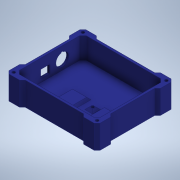
# Autodesk Inventor part: Case
Saved by Autodesk Inventor 2020 (Build 240168000, 168)
## iProperties
Created: 2020-02-03
Part Number: Case
Material: Generic
Document SubType Name: Modeling
Designer: Alex
Density: 1 g/cm^3
Appearance: Default
Author: Alex
Autodesk Inventor part; units mm, degrees
ref_plane "YZ Plane" through (0, 0, 0) normal (1, 0, 0) x (0, 1, 0)
ref_plane "XZ Plane" through (0, 0, 0) normal (0, 1, 0) x (-1, 0, 0)
ref_plane "XY Plane" through (0, 0, 0) normal (0, 0, 1) x (1, 0, 0)
sketch "Sketch1" plane through (0, 0, 0) normal (0, 1, 0) x (-1, 0, 0)
  line L0 (-60, 50) -> (-41, 50) construction
  line L1 (60, 50) -> (60, 31) construction
  line L2 (60, -50) -> (41, -50) construction
  line L3 (-60, -50) -> (-60, -31) construction
  line L4 (-60, 50) -> (60, -50) construction
  line L5 (60, 50) -> (-60, -50) construction
  line L6 (41, -50) -> (45, -54)
  line L7 (45, -54) -> (60, -54)
  line L8 (60, -54) -> (64, -50)
  line L9 (64, -50) -> (64, -35)
  line L10 (64, -35) -> (60, -31)
  line L11 (-41, -50) -> (-45, -54)
  line L12 (-45, -54) -> (-60, -54)
  line L13 (-60, -54) -> (-64, -50)
  line L14 (-64, -50) -> (-64, -35)
  line L15 (-64, -35) -> (-60, -31)
  line L16 (-60, 31) -> (-64, 35)
  line L17 (-64, 35) -> (-64, 50)
  line L18 (-64, 50) -> (-60, 54)
  line L19 (-60, 54) -> (-45, 54)
  line L20 (-45, 54) -> (-41, 50)
  line L21 (41, 50) -> (45, 54)
  line L22 (45, 54) -> (60, 54)
  line L23 (60, 54) -> (64, 50)
  line L24 (64, 50) -> (64, 35)
  line L25 (64, 35) -> (60, 31)
  line L26 (41, -50) -> (-41, -50)
  line L27 (60, -31) -> (60, -50) construction
  line L28 (60, 31) -> (60, -31)
  line L29 (41, 50) -> (60, 50) construction
  line L30 (-41, 50) -> (41, 50)
  line L31 (-60, 31) -> (-60, 50) construction
  line L32 (-41, -50) -> (-60, -50) construction
  line L33 (-60, -31) -> (-60, 31)
  point P0 (0, 0)
  point P1 (0, 0)
  point P2 (0, 0)
  dimension "d4" = 120
  dimension "d5" = 100
  dimension "d6" = 45
  dimension "d7" = 15
  dimension "d8" = 4
  dimension "d9" = 4
  dimension "d12" = 45
  dimension "d13" = 4
  constraints: 68 end point, 21 parallel, 16 perpendicular, 7 equal length, 6 collinear, 6 vertical alignment, 5 horizontal, 3 horizontal alignment, 3 midpoint, 1 coincident, 1 point on line
  measures "d4" distance of L2.start L3.start
  measures "d5" distance of L1.start L2.start
  measures "d6" angle of L6 L2
  measures "d7" distance of L6.end L7.end
  measures "d8" distance between parallel lines of L7 L2
  measures "d9" horizontal distance of L7.end L8.end
  measures "d12" angle of L2 L11
  measures "d13" distance between parallel lines of L14 L3
extrude "Extrusion2" add sketch "Sketch1" along normal blind 3
sketch "Sketch2" plane through (0, 3, 0) normal (0, 1, 0) x (1, 0, 0)
  line L0 (-64, 50) -> (-64, 35) projected
  line L1 (-64, 35) -> (-60, 31) projected
  line L2 (-60, 31) -> (-60, -31) projected
  line L3 (-60, -31) -> (-64, -35) projected
  line L4 (-64, -35) -> (-64, -50) projected
  line L5 (-64, -50) -> (-60, -54) projected
  line L6 (-60, -54) -> (-45, -54) projected
  line L7 (-45, -54) -> (-41, -50) projected
  line L8 (-41, -50) -> (41, -50) projected
  line L9 (41, -50) -> (45, -54) projected
  line L10 (45, -54) -> (60, -54) projected
  line L11 (60, -54) -> (64, -50) projected
  line L12 (64, -50) -> (64, -35) projected
  line L13 (64, -35) -> (60, -31) projected
  line L14 (60, -31) -> (60, 31) projected
  line L15 (60, 31) -> (64, 35) projected
  line L16 (64, 35) -> (64, 50) projected
  line L17 (64, 50) -> (60, 54) projected
  line L18 (60, 54) -> (45, 54) projected
  line L19 (45, 54) -> (41, 50) projected
  line L20 (41, 50) -> (-41, 50) projected
  line L21 (-41, 50) -> (-45, 54) projected
  line L22 (-45, 54) -> (-60, 54) projected
  line L23 (-60, 54) -> (-64, 50) projected
  line L24 (-42.2426, 47) -> (42.2426, 47)
  line L25 (42.2426, 47) -> (46.2426, 51) construction
  line L26 (46.2426, 51) -> (58.7574, 51) construction
  line L27 (58.7574, 51) -> (61, 48.7574) construction
  line L28 (61, 48.7574) -> (61, 36.2426) construction
  line L29 (61, 36.2426) -> (57, 32.2426) construction
  line L30 (57, 32.2426) -> (57, -32.2426)
  line L31 (57, -32.2426) -> (61, -36.2426) construction
  line L32 (61, -36.2426) -> (61, -48.7574) construction
  line L33 (61, -48.7574) -> (58.7574, -51) construction
  line L34 (58.7574, -51) -> (46.2426, -51) construction
  line L35 (46.2426, -51) -> (42.2426, -47) construction
  line L36 (42.2426, -47) -> (-42.2426, -47)
  line L37 (-42.2426, -47) -> (-46.2426, -51) construction
  line L38 (-46.2426, -51) -> (-58.7574, -51) construction
  line L39 (-58.7574, -51) -> (-61, -48.7574) construction
  line L40 (-61, -48.7574) -> (-61, -36.2426) construction
  line L41 (-61, -36.2426) -> (-57, -32.2426) construction
  line L42 (-57, -32.2426) -> (-57, 32.2426)
  line L43 (-57, 32.2426) -> (-61, 36.2426) construction
  line L44 (-61, 36.2426) -> (-61, 48.7574) construction
  line L45 (-61, 48.7574) -> (-58.7574, 51) construction
  line L46 (-58.7574, 51) -> (-46.2426, 51) construction
  line L47 (-46.2426, 51) -> (-42.2426, 47) construction
  line L48 (-42.2426, 47) -> (-52.2426, 47)
  line L49 (-52.2426, 47) -> (-57, 42.2426)
  line L50 (-57, 42.2426) -> (-57, 32.2426)
  line L51 (-57, -32.2426) -> (-57, -42.2426)
  line L52 (-57, -42.2426) -> (-52.2426, -47)
  line L53 (-52.2426, -47) -> (-42.2426, -47)
  line L54 (42.2426, -47) -> (52.2426, -47)
  line L55 (52.2426, -47) -> (57, -42.2426)
  line L56 (57, -42.2426) -> (57, -32.2426)
  line L57 (57, 32.2426) -> (57, 42.2426)
  line L58 (57, 42.2426) -> (52.2426, 47)
  line L59 (52.2426, 47) -> (42.2426, 47)
  point P0 (0, 0)
  dimension "d16" = 3
  dimension "d17" = 10
  constraints: 72 end point, 7 equal length, 4 perpendicular, 2 point on line, 1 horizontal, 1 vertical, 23 other
  measures "d16" distance between parallel lines of L20 L24
  measures "d17" distance of L24.start L48.end
extrude "Extrusion3" add sketch "Sketch2" along normal blind 30
sketch "Sketch4" plane through (0, 3, 0) normal (0, 1, 0) x (1, 0, 0)
  line L0 (45, 54) -> (41, 50) construction
  line L1 (41, 50) -> (-41, 50) construction
  line L2 (-41, 50) -> (-45, 54) construction
  line L3 (-45, 54) -> (-60, 54) construction
  line L4 (-60, 54) -> (-64, 50) construction
  line L5 (-64, 50) -> (-64, 35) construction
  line L6 (-64, 35) -> (-60, 31) construction
  line L7 (-60, 31) -> (-60, -31) construction
  line L8 (-60, -31) -> (-64, -35) construction
  line L9 (-64, -35) -> (-64, -50) construction
  line L10 (-64, -50) -> (-60, -54) construction
  line L11 (-60, -54) -> (-45, -54) construction
  line L12 (-45, -54) -> (-41, -50) construction
  line L13 (-41, -50) -> (41, -50) construction
  line L14 (41, -50) -> (45, -54) construction
  line L15 (45, -54) -> (60, -54) construction
  line L16 (60, -54) -> (64, -50) construction
  line L17 (64, -50) -> (64, -35) construction
  line L18 (64, -35) -> (60, -31) construction
  line L19 (60, -31) -> (60, 31) construction
  line L20 (60, 31) -> (64, 35) construction
  line L21 (64, 35) -> (64, 50) construction
  line L22 (64, 50) -> (60, 54) construction
  line L23 (60, 54) -> (45, 54) construction
  line L24 (-52.2426, 47) -> (52.2426, 47) construction
  line L25 (52.2426, 47) -> (57, 42.2426) construction
  line L26 (57, 42.2426) -> (57, -42.2426) construction
  line L27 (57, -42.2426) -> (52.2426, -47) construction
  line L28 (52.2426, -47) -> (-52.2426, -47) construction
  line L29 (-52.2426, -47) -> (-57, -42.2426) construction
  line L30 (-57, -42.2426) -> (-57, 42.2426) construction
  line L31 (-57, 42.2426) -> (-52.2426, 47) construction
  line L32 (-52.2426, 47) -> (-57, 42.2426) construction
  line L33 (-57, 42.2426) -> (-57, -42.2426) construction
  line L34 (-57, -42.2426) -> (-52.2426, -47) construction
  line L35 (-52.2426, -47) -> (52.2426, -47) construction
  line L36 (52.2426, -47) -> (57, -42.2426) construction
  line L37 (57, -42.2426) -> (57, 42.2426) construction
  line L38 (57, 42.2426) -> (52.2426, 47) construction
  line L39 (52.2426, 47) -> (-52.2426, 47) construction
  line L40 (-54, 9.34) -> (47.6, 9.34) construction
  line L41 (47.6, 9.34) -> (47.6, -44) construction
  line L42 (47.6, -44) -> (-54, -44) construction
  line L43 (-54, -44) -> (-54, 9.34) construction
  line L44 (9.6, -6) -> (14.6, -6)
  line L45 (14.6, -6) -> (14.6, -11)
  line L46 (14.6, -11) -> (9.6, -11)
  line L47 (9.6, -11) -> (9.6, -6)
  line L48 (9.6, -6) -> (14.6, -11) construction
  line L49 (14.6, -6) -> (9.6, -11) construction
  line L50 (45.02, -44) -> (40.02, -44)
  line L51 (40.02, -44) -> (40.02, -39)
  line L52 (40.02, -39) -> (45.02, -39)
  line L53 (45.02, -39) -> (45.02, -44)
  line L54 (45.02, -44) -> (40.02, -39) construction
  line L55 (40.02, -44) -> (45.02, -39) construction
  line L56 (-24, -0.66) -> (-4, -0.66)
  line L57 (-4, -0.66) -> (-4, -34)
  line L58 (-4, -34) -> (-24, -34)
  line L59 (-24, -34) -> (-24, -0.66)
  line L60 (21, -0.66) -> (31, -0.66)
  line L61 (31, -0.66) -> (31, -34)
  line L62 (31, -34) -> (21, -34)
  line L63 (21, -34) -> (21, -0.66)
  point P0 (-40, -41.5)
  point P1 (-38.7, 6.7)
  point P2 (12.1, -36.4)
  point P3 (12.1, -8.5)
  point P4 (36.2, 6.7)
  point P5 (42.52, -41.5)
  dimension "d20" = 53.34
  dimension "d21" = 101.6
  dimension "d23" = 3
  dimension "d24" = 3
  dimension "d25" = 14
  dimension "d26" = 1.3
  dimension "d27" = 50.8
  dimension "d29" = 2.5
  dimension "d30" = 5.1
  dimension "d31" = 27.9
  dimension "d32" = 15.2
  dimension "d33" = 24.1
  dimension "d34" = 96.52
  dimension "d35" = 30
  dimension "d36" = 50
  dimension "d37" = 10
  dimension "d38" = 10
  dimension "d39" = 75
  dimension "d40" = 85
  dimension "d41" = 5
  constraints: 48 end point, 10 parallel, 5 horizontal, 5 perpendicular, 4 midpoint, 3 equal length, 2 collinear, 2 horizontal alignment, 1 vertical alignment
  measures "d20" distance of L40.end L41.end
  measures "d21" distance of L40.start L40.end
  measures "d23" distance between parallel lines of L42 L28
  measures "d24" distance between parallel lines of L30 L43
  measures "d25" distance from line of point (-40, -41.5) L43
  measures "d26" horizontal distance of point (-38.7, 6.7) point (-40, -41.5)
  measures "d27" horizontal distance of point (12.1, -8.5) point (-38.7, 6.7)
  measures "d29" distance from line of point (42.52, -41.5) L42
  measures "d30" vertical distance of point (12.1, -36.4) point (-40, -41.5)
  measures "d31" distance of point (12.1, -8.5) point (12.1, -36.4)
  measures "d32" vertical distance of point (36.2, 6.7) point (12.1, -8.5)
  measures "d33" horizontal distance of point (36.2, 6.7) point (12.1, -8.5)
  measures "d34" distance from line of point (42.52, -41.5) L43
  measures "d35" distance between parallel lines of L59 L43
  measures "d36" distance between parallel lines of L57 L43
  measures "d37" distance between parallel lines of L56 L40
  measures "d38" distance between parallel lines of L58 L42
  measures "d39" distance between parallel lines of L63 L43
  measures "d40" distance between parallel lines of L61 L43
  measures "d41" distance of L45.end L46.end
extrude "Extrusion4" add sketch "Sketch4" along normal blind 3
chamfer "Chamfer1" distance 3 angle 45 16 edges at (-14, 3, 34) (-4, 3, 17.33) (21, 3, 17.33) (-24, 3, 17.33) (26, 3, 34) (40.02, 3, 41.5) (42.52, 3, 39) (45.02, 3, 41.5) (42.52, 3, 44) (9.6, 3, 8.5) (12.1, 3, 11) (14.6, 3, 8.5) (12.1, 3, 6) (26, 3, 0.66) (-14, 3, 0.66) (31, 3, 17.33)
sketch "Sketch5" plane through (0, 6, 0) normal (0, 1, 0) x (1, 0, 0)
  line L0 (14.6, -11) -> (14.6, -6) construction
  line L1 (14.6, -6) -> (9.6, -6) construction
  line L2 (9.6, -6) -> (9.6, -11) construction
  line L3 (9.6, -11) -> (14.6, -11) construction
  line L4 (40.02, -44) -> (45.02, -44) construction
  line L5 (45.02, -44) -> (45.02, -39) construction
  line L6 (45.02, -39) -> (40.02, -39) construction
  line L7 (40.02, -39) -> (40.02, -44) construction
  point P0 (0, 0)
  point P1 (12.1, -8.5)
  point P2 (42.52, -41.5)
  point P3 (14.6, -8.5)
  point P4 (45.02, -41.5)
  point P5 (12.1, -6)
  point P6 (42.52, -39)
  constraints: 4 midpoint, 2 horizontal alignment, 2 vertical alignment
hole "Hole1" at (12.1, 6, 8.5) at (42.52, 6, 41.5) direction (0, -1, 0) diameter 4 depth 5
sketch "Sketch6" plane through (-57, 3, 42.2426) normal (1, 0, 0) x (0, 0, -1)
  line L0 (44.5826, 0) -> (5.2426, 0) construction
  line L1 (5.2426, 0) -> (44.5826, 0) construction
  line L2 (5.2426, 0) -> (44.5826, 0) construction
  line L3 (44.5826, 0) -> (5.2426, 0) construction
  line L4 (-4.7574, 0) -> (6.2426, 0) construction
  line L5 (-4.7574, 0) -> (0, 0) construction
  line L6 (0, 0) -> (84.4853, 0) construction
  line L7 (84.4853, 0) -> (89.2426, 0) construction
  line L8 (89.2426, 0) -> (84.4853, 0) construction
  line L9 (84.4853, 0) -> (0, 0) construction
  line L10 (0, 0) -> (-4.7574, 0) construction
  line L11 (6.2426, 0) -> (-4.7574, 0) construction
  line L12 (39.2426, 0) -> (28.2426, 0) construction
  line L13 (28.2426, 0) -> (39.2426, 0) construction
  line L14 (-1.7574, 0) -> (51.5826, 0) construction
  line L15 (41.5826, 3) -> (8.2426, 3) construction
  line L16 (8.2426, 3) -> (41.5826, 3) construction
  line L17 (41.5826, 3) -> (44.5826, 0) construction
  line L18 (44.5826, 0) -> (41.5826, 3) construction
  line L19 (8.2426, 3) -> (5.2426, 0) construction
  line L20 (8.2426, 3) -> (5.2426, 0) construction
  line L21 (84.4853, 0) -> (0, 0) construction
  line L22 (84.4853, 0) -> (84.4853, 30) construction
  line L23 (0, 30) -> (84.4853, 30) construction
  line L24 (0, 0) -> (0, 30) construction
  line L25 (29.8326, 16.2) -> (42.3326, 16.2)
  line L26 (42.3326, 16.2) -> (42.3326, 4.7)
  line L27 (42.3326, 4.7) -> (29.8326, 4.7)
  line L28 (29.8326, 4.7) -> (29.8326, 16.2)
  point P0 (42.2426, -3)
  dimension "d55" = 11.5
  dimension "d56" = 12.5
  dimension "d57" = 1.7
  dimension "d58" = 9.25
  constraints: 8 end point, 2 parallel, 1 horizontal, 1 perpendicular, 1 other
  measures "d55" distance between parallel lines of L25 L27
  measures "d56" distance between parallel lines of L26 L28
  measures "d57" distance between parallel lines of L27 L15
  measures "d58" distance from line of point (51.583, 0) L26
extrude "Extrusion5" cut sketch "Sketch6" against normal blind 10
sketch "Sketch7" plane through (0, 33, 0) normal (0, 1, 0) x (1, 0, 0)
  line L0 (41, -50) -> (45, -54) construction
  line L1 (45, -54) -> (60, -54) construction
  line L2 (60, -54) -> (64, -50) construction
  line L3 (64, -50) -> (64, -35) construction
  line L4 (64, -35) -> (60, -31) construction
  line L5 (60, -31) -> (60, 31) construction
  line L6 (60, 31) -> (64, 35) construction
  line L7 (64, 35) -> (64, 50) construction
  line L8 (64, 50) -> (60, 54) construction
  line L9 (60, 54) -> (45, 54) construction
  line L10 (45, 54) -> (41, 50) construction
  line L11 (41, 50) -> (-41, 50) construction
  line L12 (-41, 50) -> (-45, 54) construction
  line L13 (-45, 54) -> (-60, 54) construction
  line L14 (-60, 54) -> (-64, 50) construction
  line L15 (-64, 50) -> (-64, 35) construction
  line L16 (-64, 35) -> (-60, 31) construction
  line L17 (-60, 31) -> (-60, -31) construction
  line L18 (-60, -31) -> (-64, -35) construction
  line L19 (-64, -35) -> (-64, -50) construction
  line L20 (-64, -50) -> (-60, -54) construction
  line L21 (-60, -54) -> (-45, -54) construction
  line L22 (-45, -54) -> (-41, -50) construction
  line L23 (-41, -50) -> (41, -50) construction
  line L24 (52.2426, -47) -> (-52.2426, -47) construction
  line L25 (-52.2426, -47) -> (-57, -42.2426) construction
  line L26 (-57, -42.2426) -> (-57, 42.2426) construction
  line L27 (-57, 42.2426) -> (-52.2426, 47) construction
  line L28 (-52.2426, 47) -> (52.2426, 47) construction
  line L29 (52.2426, 47) -> (57, 42.2426) construction
  line L30 (57, 42.2426) -> (57, -42.2426) construction
  line L31 (57, -42.2426) -> (52.2426, -47) construction
  line L32 (-64, -35) -> (-64, -50) construction
  line L33 (-57, -42.2426) -> (-52.2426, -47) construction
  line L34 (-64, -50) -> (-52.2426, -47) construction
  line L35 (-60, -54) -> (-45, -54) construction
  line L36 (-57, -42.2426) -> (-57, 42.2426) construction
  line L37 (-60, -54) -> (-57, -42.2426) construction
  line L38 (-57, 0) -> (57, 0) construction
  line L39 (57, -42.2426) -> (57, 42.2426) projected
  line L40 (-52.2426, -47) -> (37.02, -47) projected
  line L41 (0, -50) -> (0, 50) construction
  line L42 (41, 50) -> (-41, 50) projected
  point P0 (0, 0)
  point P1 (-58.6297, -48.6297)
  point P2 (58.6297, -48.6297)
  point P3 (-58.6297, 48.6297)
  point P4 (58.6297, 48.6297)
  constraints: 8 end point, 4 midpoint, 3 symmetric about line, 2 point on line
hole "Hole2" at (-58.6297, 33, 48.6297) at (58.6297, 33, 48.6297) at (58.6297, 33, -48.6297) at (-58.6297, 33, -48.6297) direction (0, -1, 0) diameter 4 depth 5
sketch "Sketch8" plane through (-60, 0, -31) normal (-1, 0, 0) x (0, 0, 1)
  line L0 (30.91, 7.7) -> (30.91, 19.2) construction
  line L1 (30.91, 19.2) -> (43.41, 19.2) construction
  line L2 (43.41, 19.2) -> (43.41, 7.7) construction
  line L3 (43.41, 7.7) -> (30.91, 7.7) construction
  line L4 (0, 0) -> (62, 0) construction
  line L5 (62, 0) -> (62, 33) construction
  line L6 (0, 33) -> (62, 33) construction
  line L7 (0, 0) -> (0, 33) construction
  line L8 (30.91, 19.2) -> (30.91, 7.7) construction
  line L9 (30.91, 7.7) -> (43.41, 7.7) construction
  line L10 (43.41, 7.7) -> (43.41, 19.2) construction
  line L11 (43.41, 19.2) -> (30.91, 19.2) construction
  line L12 (-11.2426, 3) -> (73.2426, 3) construction
  line L13 (-11.2426, 3) -> (-11.2426, 33) construction
  line L14 (73.2426, 33) -> (-11.2426, 33) construction
  line L15 (73.2426, 3) -> (73.2426, 33) construction
  arc A0 (11.5, 24.8741) -> (14.5, 24.8741) centre (13, 16) ccw
  circle A1 centre (13, 16) radius 10 construction
  line L16 (11.5, 25.8869) -> (11.5, 6.1131) construction
  line L17 (14.5, 25.8869) -> (14.5, 6.1131) construction
  line L18 (11.5, 16) -> (13, 16) construction
  line L19 (13, 16) -> (14.5, 16) construction
  line L20 (11.5, 24.8741) -> (11.5, 25.8869)
  line L21 (14.5, 24.8741) -> (14.5, 25.8869)
  arc A2 (14.5, 24.8741) -> (11.5, 24.8741) centre (13, 16) ccw construction
  arc A3 (14.5, 25.8869) -> (11.5, 25.8869) centre (13, 16) ccw
  point P0 (31, 0)
  dimension "d68" = 18
  dimension "d69" = 20
  dimension "d70" = 3
  dimension "d71" = 13
  dimension "d72" = 13
  constraints: 12 end point, 10 point on circle, 4 centre point, 3 collinear, 2 coincident, 2 midpoint, 2 point on line, 2 vertical, 1 horizontal
  measures "d68" diameter of A0
  measures "d69" diameter of A1
  measures "d70" distance between parallel lines of L16 L17
  measures "d71" distance from line of L12 A0.centre
  measures "d72" distance from line of L7 A0.centre
extrude "Extrusion6" cut sketch "Sketch8" against normal blind 10
sketch "Sketch9" plane through (41, 0, -50) normal (0, 0, -1) x (-1, 0, 0)
  point P0 (41, 0)
equation "\"d9\" = d8"
equation "\"d13\" = d9"
body "Solid2"
